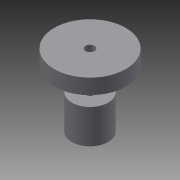
# Autodesk Inventor part: motor
Saved by Autodesk Inventor 2015 (Build 190159000, 159)
## iProperties
Created: 2015-03-03
Part Number: motor
Material: Generic
Document SubType Name: Modeling
Designer: Qiuyang
Density: 1 g/cm^3
Appearance: Default
Author: Qiuyang
Autodesk Inventor part; units mm, degrees
ref_plane "YZ Plane" through (0, 0, 0) normal (1, 0, 0) x (0, 1, 0)
ref_plane "XZ Plane" through (0, 0, 0) normal (0, 1, 0) x (-1, 0, 0)
ref_plane "XY Plane" through (0, 0, 0) normal (0, 0, 1) x (1, 0, 0)
sketch "Sketch1" plane through (0, 0, 0) normal (0, 1, 0) x (-1, 0, 0)
  circle A0 centre (0, 0) radius 15.24
  dimension "d0" = 30.48
  constraints: 1 centre point, 1 coincident
  measures "d0" diameter of A0
extrude "Extrusion1" add sketch "Sketch1" along normal blind 28.575
sketch "Sketch2" plane through (0, 28.575, 0) normal (0, 1, 0) x (1, 0, 0)
  circle A0 centre (0, 0) radius 3.81
  dimension "d3" = 7.62
  constraints: 1 centre point, 1 coincident
  measures "d3" diameter of A0
extrude "Extrusion2" add sketch "Sketch2" along normal blind 19.05
sketch "Sketch3" plane through (0, 47.625, 0) normal (0, 1, 0) x (1, 0, 0)
  circle A0 centre (0, 0) radius 3.81 projected
  circle A1 centre (0, 0) radius 30.0101
  dimension "d6" = 60.0202
  constraints: 1 centre point, 1 coincident
  measures "d6" diameter of A1
extrude "Extrusion3" add sketch "Sketch3" along normal blind 12.7
body "Solid1"
